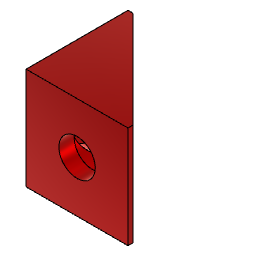
kostkav2 v3 (Autodesk Fusion 360 design; units mm, degrees)
Autodesk Fusion 360 part; units mm, degrees
sketch "Sketch1" plane through (0, 0, 0) normal (0, 1, 0) x (1, 0, 0)
  line L0 (0, 0) -> (20, 0)
  line L1 (20, 0) -> (20, -20)
  line L2 (20, -20) -> (0, -20)
  line L3 (0, -20) -> (0, 0)
  dimension "d2" = 20
  dimension "d3" = 20
  constraint horizontal L0
  constraint vertical L1
  constraint horizontal L2
  constraint vertical L3
  constraint coincident L0.start L3.end
  measures "d2" distance of L0.start L0.end
  measures "d3" distance of L0.start L2.end
extrude "Extrude4" add sketch "Sketch1" along normal blind 20 makes body 1
extrude "Extrude1" add sketch "Sketch1" along normal blind 20 separate body makes body 2
sketch "Sketch2" plane through (0, 20, 0) normal (0, 1, 0) x (-1, 0, 0)
  line L0 (0, 20) -> (-20, 20)
  line L1 (-20, 20) -> (-20, 0)
  line L2 (-20, 0) -> (0, 0)
  line L3 (0, 0) -> (0, 20)
  line L4 (-20, 20) -> (0, 0) construction
  line L5 (0, 20) -> (-20, 0) construction
  circle A0 centre (-10, 10) radius 3.57
  circle A1 centre (-10, 10) radius 5.5
  dimension "d6" = 7.14
  dimension "d19" = 11
  constraint coincident L0.end L1.start
  constraint coincident L2.end L3.start
  constraint coincident L0.start L3.end
  constraint coincident L1.end L2.start
  constraint midpoint L5 A0.centre
  constraint concentric A0 A1
  measures "d6" diameter of A0
  measures "d19" diameter of A1
sketch "Sketch5" plane through (0, 0, 0) normal (-1, 0, 0) x (0, -1, 0)
  line L0 (0, 0) -> (0, 20)
  line L1 (0, 20) -> (-20, 20)
  line L2 (-20, 20) -> (-20, 0)
  line L3 (-20, 0) -> (0, 0)
sketch "Sketch6" plane through (20, 0, 0) normal (1, 0, 0) x (0, 1, 0)
  line L0 (0, 20) -> (0, 0)
  line L1 (0, 0) -> (20, 0)
  line L2 (20, 0) -> (20, 20)
  line L3 (20, 20) -> (0, 20)
  line L4 (0, 20) -> (20, 0) construction
  line L5 (20, 20) -> (0, 0) construction
  circle A0 centre (10, 10) radius 3.57
  circle A1 centre (10, 10) radius 5.5
  dimension "d14" = 7.14
  dimension "d20" = 11
  constraint coincident L0.start L3.end
  constraint coincident L1.end L2.start
  constraint coincident L2.end L3.start
  constraint coincident L0.end L1.start
  constraint midpoint L4 A0.centre
  constraint concentric A0 A1
  measures "d14" diameter of A0
  measures "d20" diameter of A1
extrude "Extrude5" cut sketch "Sketch6" against normal blind 20 contours A0 bodies 1 2
extrude "Extrude6" cut sketch "Sketch2" against normal blind 20 contours A0 bodies 1 2
extrude "Extrude7" cut sketch "Sketch2" against normal blind 16.97 contours A1 bodies 1 2
extrude "Extrude8" cut sketch "Sketch6" against normal blind 16.97 contours A1 bodies 1 2
sketch "Sketch8" plane through (0, 0, 20) normal (0, 0, 1) x (-1, 0, 0)
  line L0 (0, 0) -> (-20, 0)
  line L1 (-20, 0) -> (-20, -20)
  line L2 (-20, -20) -> (0, -20)
  line L3 (0, -20) -> (0, 0)
  line L4 (-20, 0) -> (-19, 0)
  line L5 (0, -20) -> (0, -19)
  line L6 (-20, 0) -> (-20, -1)
  line L7 (0, -20) -> (-1, -20)
  line L8 (-1, -20) -> (-20, -1)
  dimension "d27" = 1
  dimension "d28" = 1
  dimension "d29" = 1
  dimension "d30" = 1
  constraint coincident L0.end L1.start
  constraint perpendicular L1 L4
  constraint coincident L2.end L3.start
  constraint perpendicular L2 L5
  constraint perpendicular L4 L6
  constraint perpendicular L5 L7
  measures "d27" distance of L0.end L4.end
  measures "d28" distance of L2.end L5.end
  measures "d29" distance of L0.end L6.end
  measures "d30" distance of L2.end L7.end
extrude "Extrude9" cut sketch "Sketch8" against normal blind 21 contours L1 L2 L8 bodies 1 2
sketch "Sketch3" plane through (0, 0, 0) normal (1, 0, 0) x (0, 1, 0)
sketch "Sketch4" plane through (0, 0, 0) normal (-1, 0, 0) x (0, -1, 0)
  line L0 (0, 0) -> (0, 20)
  line L1 (0, 20) -> (-20, 20)
  line L2 (-20, 20) -> (-20, 0)
  line L3 (-20, 0) -> (0, 0)
  line L4 (0, 0) -> (-20, 20) construction
  line L5 (0, 20) -> (-20, 0) construction
  circle A0 centre (-10, 10) radius 3.57
  dimension "d7" = 7.14
  constraint coincident L0.start L3.end
  constraint coincident L1.end L2.start
  constraint coincident L0.end L1.start
  constraint coincident L2.end L3.start
  constraint midpoint L4 A0.centre
  measures "d7" diameter of A0
extrude "Extrude2" [suppressed]
extrude "Extrude3" [suppressed]
hidden bodies 1
equation "w = 20 mm"
named bodies: "Kostka"
